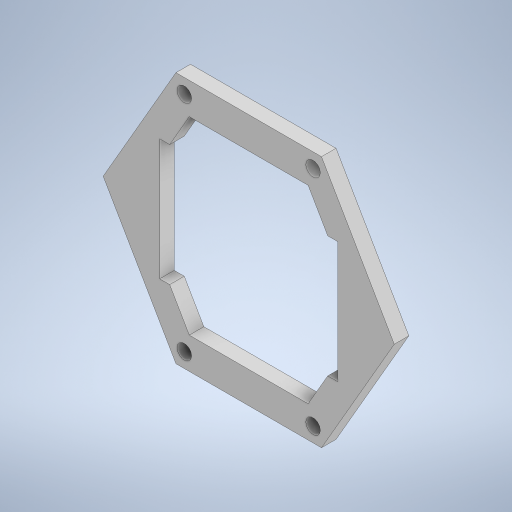
# Autodesk Inventor part: ArmDriverBoard
Saved by Autodesk Inventor 2023 (Build 270158000, 158)
## iProperties
Created: 2023-11-22
Part Number: ArmDriverBoard
Material: Generic
Document SubType Name: Modeling
Designer: LattePanda
Density: 1 g/cm^3
Appearance: Default
Author: LattePanda
Autodesk Inventor part; units mm, degrees
ref_plane "YZ Plane" through (0, 0, 0) normal (1, 0, 0) x (0, 1, 0)
ref_plane "XZ Plane" through (0, 0, 0) normal (0, 1, 0) x (-1, 0, 0)
ref_plane "XY Plane" through (0, 0, 0) normal (0, 0, 1) x (1, 0, 0)
sketch "Base" plane through (0, 0, 0) normal (0, 0, 1) x (1, 0, 0)
  line L0 (-29.9999, 0.0001) -> (-15, -25.9807)
  line L1 (15, -25.9808) -> (30, 0)
  line L2 (-15, -25.9807) -> (15, -25.9808)
  line L3 (30, 0) -> (15, 25.9808)
  line L4 (15, 25.9808) -> (-15, 25.9808)
  line L5 (-15, 25.9808) -> (-30, 0)
  line L6 (0, 25.9808) -> (0, -25.9808) construction
  line L7 (-30, 0) -> (30, 0) construction
  line L8 (-24.8039, 3) -> (-13.268, 22.9808) construction
  line L9 (-13.268, 22.9808) -> (13.2679, 22.9808) construction
  line L10 (13.2679, 22.9808) -> (24.8038, 3) construction
  line L11 (24.8038, 3) -> (-24.8039, 3) construction
  circle A0 centre (-13.268, 22.9808) radius 1.5
  circle A1 centre (13.2679, 22.9808) radius 1.5
  circle A2 centre (-24.8039, 0) radius 1.5 construction
  line L12 (-24.8039, 3) -> (-26.5359, 0) construction
  circle A3 centre (24.8039, 0.0001) radius 1.5 construction
  circle A4 centre (-13.268, -22.9808) radius 1.5
  circle A5 centre (13.2679, -22.9808) radius 1.5
  point P0 (0, 0)
  point P1 (0, 0)
  point P2 (-30, 0.0001)
  dimension "d1" = 30
  dimension "d6" = 120
  dimension "d7" = 120
  dimension "d8" = 120
  dimension "d9" = 120
  dimension "d10" = 120
  dimension "d13" = 3
  dimension "d14" = 3
  dimension "d15" = 3
  constraints: 26 end point, 6 centre point, 5 equal length, 3 coincident, 3 midpoint, 3 symmetric about line, 2 point on line, 1 collinear, 1 equal radius, 1 horizontal, 1 tangent, 6 other
  measures "d1" distance of L3.end L4.end
  measures "d6" angle of L4 L5
  measures "d7" angle of L3 L4
  measures "d8" angle of L0 L5
  measures "d9" angle of L1 L3
  measures "d10" angle of L2 L0
  measures "d13" distance between parallel lines of L5 L8
  measures "d14" diameter of A0
  measures "d15" diameter of A1
extrude "BaseFeature" add sketch "Base" along normal blind 3
sketch "DriverProfile" plane through (0, 0, 3) normal (0, 0, 1) x (1, 0, 0)
  line L0 (-42, 0) -> (42, 0) construction
  line L1 (0, -36.3731) -> (0, 36.3731) construction
  line L2 (-21, 21.5) -> (21, 21.5)
  line L3 (21, 21.5) -> (21, -21.5)
  line L4 (21, -21.5) -> (-21, -21.5)
  line L5 (-21, -21.5) -> (-21, 21.5)
  line L6 (19, 19.5) -> (-19, 19.5) construction
  line L7 (-19, 19.5) -> (-19, -19.5) construction
  line L8 (-19, -19.5) -> (19, -19.5) construction
  line L9 (19, -19.5) -> (19, 19.5) construction
  circle A0 centre (-17.375, 17.875) radius 1.625
  circle A1 centre (17.375, 17.875) radius 1.625
  circle A2 centre (-17.375, -17.875) radius 1.625
  circle A3 centre (17.375, -17.875) radius 1.625
  line L10 (-18.35, 12.5) -> (18.35, 12.5)
  line L11 (18.35, 12.5) -> (18.35, -12.5)
  line L12 (18.35, -12.5) -> (-18.35, -12.5)
  line L13 (-18.35, -12.5) -> (-18.35, 12.5)
  point P0 (0, 0)
  point P1 (0, 21.5)
  point P2 (-21, 0)
  point P3 (0, 12.5)
  point P4 (-18.35, 0)
  dimension "d16" = 43
  dimension "d17" = 42
  dimension "d18" = 2
  dimension "d19" = 3.25
  dimension "d20" = 36.7
  dimension "d21" = 25
  constraints: 24 end point, 6 parallel, 4 centre point, 4 midpoint, 4 point on line, 3 perpendicular, 3 symmetric about line, 2 horizontal, 2 tangent, 6 other
  measures "d16" distance of L4.end L2.start
  measures "d17" distance of L2.start L2.end
  measures "d18" distance between parallel lines of L2 L6
  measures "d19" diameter of A0
  measures "d20" distance of L11.end L12.end
  measures "d21" distance between parallel lines of L12 L10
extrude "HeatsinkFeature" cut sketch "DriverProfile" against normal through all contours L10 L11 L12 L13
sketch "Contacts" plane through (0, 0, 3) normal (0, 0, 1) x (1, 0, 0)
  circle A0 centre (17.375, -17.875) radius 3.625 construction
  circle A1 centre (17.375, -17.875) radius 1.625 projected
  line L0 (18.35, -12.5) -> (-18.35, -12.5) construction
  line L1 (16.2925, -12.5) -> (12.251, -19.5)
  line L2 (15, -25.9808) -> (30, 0) construction
  line L3 (-19, -19.5) -> (19, -19.5) construction
  line L4 (12.251, -19.5) -> (0, -19.5)
  line L5 (0, -36.3731) -> (0, 36.3731) construction
  line L6 (-16.2925, -12.5) -> (-12.251, -19.5)
  line L7 (-12.251, -19.5) -> (0, -19.5)
  line L8 (-42, 0) -> (42, 0) construction
  line L9 (16.2925, 12.5) -> (12.251, 19.5)
  line L10 (12.251, 19.5) -> (0, 19.5)
  line L11 (-12.251, 19.5) -> (0, 19.5)
  line L12 (-16.2925, 12.5) -> (-12.251, 19.5)
  line L13 (-16.2925, -12.5) -> (16.2925, -12.5)
  line L14 (16.2925, 12.5) -> (-16.2925, 12.5)
  line L15 (-18.35, 12.5) -> (18.35, 12.5) projected
  point P0 (0, 0)
  dimension "d24" = 2
  constraints: 20 end point, 7 symmetric about line, 2 collinear, 2 point on line, 1 centre point, 1 coincident, 1 midpoint, 1 parallel, 1 tangent
  measures "d24" radial gap between concentric circles of A0 A1
extrude "ContactsFeature" cut sketch "Contacts" against normal through all contours L1 L4 L7 L6 L13 | L14 L12 L11 L10 L9
equation "\"d7\" = d6"
equation "\"d8\" = d6"
equation "\"d9\" = d6"
equation "\"d10\" = d6"
body "Solid1"
